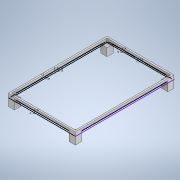
# Autodesk Inventor part: 底座
Saved by Autodesk Inventor 2022.5 (Build 265521000, 521)
## iProperties
Created: 2025-01-08
Part Number: 底座
Material: 常规
Document SubType Name: Modeling
Designer: Administrator
Density: 1 g/cm^3
Appearance: 默认
Mass: 5.085 g
Surface Area: 61.98 cm^2
Volume: 5.085 cm^3
Author: Administrator
Autodesk Inventor part; units mm, degrees
ref_plane "YZ Plane" through (0, 0, 0) normal (1, 0, 0) x (0, 1, 0)
ref_plane "XZ Plane" through (0, 0, 0) normal (0, 1, 0) x (-1, 0, 0)
ref_plane "XY Plane" through (0, 0, 0) normal (0, 0, 1) x (1, 0, 0)
sketch "草图1" plane through (0, 0, 0) normal (0, 1, 0) x (-1, 0, 0)
  line L0 (0, 0) -> (83, 0)
  line L1 (83, 0) -> (83, -124)
  line L2 (83, -124) -> (0, -124)
  line L3 (0, -124) -> (0, 0)
  line L4 (-2, 2) -> (85, 2)
  line L5 (85, 2) -> (85, -126)
  line L6 (85, -126) -> (-2, -126)
  line L7 (-2, -126) -> (-2, 2)
  dimension "d0" = 83
  dimension "d1" = 124
  dimension "d2" = 2
  dimension "d3" = 2
  dimension "d4" = 2
  constraints: 16 end point, 4 parallel, 2 horizontal, 2 perpendicular
  measures "d0" distance of L1.end L2.end
  measures "d1" distance of L0.end L1.end
  measures "d2" distance between parallel lines of L2 L6
  measures "d3" distance between parallel lines of L1 L5
  measures "d4" distance between parallel lines of L0 L4
extrude "拉伸1" add sketch "草图1" along normal blind 5 contours L0 L1 L2 L3 | L4 L5 L6 L7
sketch "草图2" plane through (-85, 0, 2) normal (0, 0, 1) x (1, 0, 0)
  line L0 (0, 0) -> (87, 0) projected
  line L1 (87, 0) -> (87, 5) projected
  line L2 (0, 5) -> (87, 5) projected
  line L3 (0, 0) -> (0, 5) projected
  line L4 (85, 0) -> (2, 0) projected
  line L5 (8, 0) -> (79, 0)
  line L6 (79, 0) -> (79, 2.5)
  line L7 (79, 2.5) -> (8, 2.5)
  line L8 (8, 2.5) -> (8, 0)
  point P0 (79, 1.25)
  dimension "d8" = 8
  dimension "d9" = 8
  constraints: 8 end point, 2 parallel, 1 horizontal, 1 midpoint, 1 perpendicular, 1 point on line
  measures "d8" distance between parallel lines of L3 L8
  measures "d9" distance from line of L1 point (79, 1.25)
extrude "拉伸2" cut sketch "草图2" against normal through all contours L8 L7 L6 L0
sketch "草图3" plane through (2, 0, 2) normal (1, 0, 0) x (0, 0, -1)
  line L0 (2, 0) -> (126, 0) projected
  line L1 (8, 0) -> (120, 0)
  line L2 (120, 0) -> (120, 2.5)
  line L3 (120, 2.5) -> (8, 2.5)
  line L4 (8, 2.5) -> (8, 0)
  line L5 (0, 0) -> (0, 5) projected
  line L6 (128, 0) -> (128, 5) projected
  line L7 (0, 5) -> (128, 5) projected
  point P0 (8, 1.25)
  point P1 (120, 1.25)
  dimension "d12" = 8
  dimension "d13" = 8
  dimension "d14" = 2.5
  constraints: 8 end point, 2 midpoint, 2 parallel, 1 horizontal, 1 perpendicular, 1 point on line
  measures "d12" distance from line of L5 point (8, 1.25)
  measures "d13" distance from line of L6 point (120, 1.25)
  measures "d14" distance between parallel lines of L7 L3
extrude "拉伸3" cut sketch "草图3" against normal through all
sketch "草图4" plane through (0, 0, 0) normal (0, -1, 0) x (1, 0, 0)
  line L0 (-6, -6) -> (2, -6) projected
  line L1 (2, 2) -> (2, -6) projected
  line L2 (-6, 2) -> (2, 2) projected
  line L3 (-6, 2) -> (-6, -6) projected
  line L4 (-6, -6) -> (2, -6) projected
  line L5 (-77, -126) -> (-77, -118) projected
  line L6 (-85, 2) -> (-77, 2) projected
  line L7 (-85, -6) -> (-85, 2) projected
  line L8 (2, -118) -> (-6, -118) projected
  line L9 (-85, -126) -> (-85, -118) projected
  line L10 (-77, -126) -> (-85, -126) projected
  line L11 (-77, -126) -> (-77, -118) projected
  line L12 (2, -118) -> (-6, -118) projected
  line L13 (-6, 2) -> (-6, -6) projected
  line L14 (2, -126) -> (-6, -126) projected
  line L15 (2, -118) -> (2, -126) projected
  line L16 (-6, -118) -> (-6, -126) projected
  line L17 (-77, -118) -> (-85, -118) projected
  line L18 (-85, -126) -> (-85, -118) projected
  line L19 (-77, -126) -> (-85, -126) projected
  line L20 (-77, -126) -> (-77, -118) projected
  line L21 (-6, -6) -> (2, -6) projected
  line L22 (2, 2) -> (2, -6) projected
  line L23 (-6, 2) -> (2, 2) projected
  line L24 (-6, -6) -> (2, -6) projected
  line L25 (-85, 2) -> (-77, 2) projected
  line L26 (-85, -6) -> (-85, 2) projected
  line L27 (-6, 2) -> (-6, -6) projected
  line L28 (2, -126) -> (-6, -126) projected
  line L29 (2, -118) -> (2, -126) projected
  line L30 (-77, -118) -> (-85, -118) projected
  line L31 (-77, -6) -> (-77, 2) projected
  line L32 (-85, -6) -> (-77, -6) projected
  line L33 (2, -118) -> (-6, -118) projected
  line L34 (-85, -126) -> (-85, -118) projected
  line L35 (-77, -126) -> (-85, -126) projected
  line L36 (-77, -6) -> (-77, 2) projected
  line L37 (2, 2) -> (2, -6) projected
  line L38 (-6, 2) -> (2, 2) projected
  line L39 (-6, 2) -> (-6, -6) projected
  line L40 (-85, -6) -> (-77, -6) projected
  line L41 (-77, -126) -> (-77, -118) projected
  line L42 (-85, 2) -> (-77, 2) projected
  line L43 (-85, -6) -> (-85, 2) projected
  line L44 (2, -118) -> (-6, -118) projected
  line L45 (-6, -118) -> (-6, -126) projected
  line L46 (2, -126) -> (-6, -126) projected
  line L47 (2, -118) -> (2, -126) projected
  line L48 (-85, -6) -> (-77, -6) projected
  line L49 (-77, -6) -> (-77, 2) projected
  line L50 (-85, 2) -> (-77, 2) projected
  line L51 (-85, -6) -> (-85, 2) projected
  line L52 (2, 2) -> (2, -6) projected
  line L53 (-6, 2) -> (2, 2) projected
  line L54 (-85, -6) -> (-77, -6) projected
  line L55 (-6, -118) -> (-6, -126) projected
  line L56 (-77, -118) -> (-85, -118) projected
  line L57 (-6, -118) -> (-6, -126) projected
  line L58 (2, -126) -> (-6, -126) projected
  line L59 (2, -118) -> (2, -126) projected
  line L60 (-77, -6) -> (-77, 2) projected
  line L61 (-77, -118) -> (-85, -118) projected
  line L62 (-85, -126) -> (-85, -118) projected
  line L63 (-77, -126) -> (-85, -126) projected
  point P0 (0, 0)
extrude "拉伸4" add sketch "草图4" along normal blind 10
extrude "拉伸5" cut sketch "草图1" along normal blind 43 contours L0 L1 L2 L3
